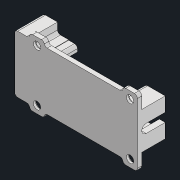
# Autodesk Inventor part: SyringeCasing
Saved by Autodesk Inventor 2022.2 (Build 262287010, 287A)
## iProperties
Created: 2022-06-05
Part Number: SyringeCasing
Material: Generic
Document SubType Name: Modeling
Designer: frede
Density: 1 g/cm^3
Appearance: Default
Author: frede
Autodesk Inventor part; units mm, degrees
ref_plane "YZ Plane" through (0, 0, 0) normal (1, 0, 0) x (0, 1, 0)
ref_plane "XZ Plane" through (0, 0, 0) normal (0, 1, 0) x (-1, 0, 0)
ref_plane "XY Plane" through (0, 0, 0) normal (0, 0, 1) x (1, 0, 0)
sketch "Sketch1" plane through (0, 0, 0) normal (0, 0, 1) x (1, 0, 0)
  line L0 (-75.5, -15.5) -> (-73.5, -15.5) construction
  line L1 (-75.5, 15.5) -> (-73.5, 15.5) construction
  line L2 (-75.5, 15.5) -> (-75.5, 10.4021) construction
  line L3 (-75.5, 10.4021) -> (-75.5, 3.3083) construction
  line L4 (-75.5, 3.3083) -> (-75.5, -3.3083) construction
  line L5 (-75.5, -3.3083) -> (-75.5, -10.4021) construction
  line L6 (-75.5, -10.4021) -> (-75.5, -15.5) construction
  line L7 (-73.5, -15.5) -> (-73.5, -10.4021) construction
  line L8 (-73.5, 10.4021) -> (-73.5, 15.5) construction
  line L9 (-73.5, -8.85) -> (-65.9, -8.85) construction
  line L10 (-73.5, 8.85) -> (-65.9, 8.85) construction
  line L11 (0, 8.575) -> (0, -8.575) construction
  line L12 (0, -8.575) -> (-65.9, -8.575) construction
  line L13 (0, 8.575) -> (-65.9, 8.575) construction
  line L14 (-65.9, 8.575) -> (-65.9, 8.85) construction
  line L15 (-65.9, -8.85) -> (-65.9, -8.575) construction
  line L16 (-73.5, -10.4021) -> (-73.5, -8.85) construction
  line L17 (-73.5, 8.85) -> (-73.5, 10.4021) construction
  line L18 (-65.8, 8.675) -> (0.1, 8.675)
  line L19 (0.1, 8.675) -> (0.1, -8.675)
  line L20 (0.1, -8.675) -> (-65.8, -8.675)
  line L21 (-65.8, -8.675) -> (-65.8, -8.95)
  line L22 (-65.8, -8.95) -> (-73.4, -8.95)
  line L23 (-73.4, -8.95) -> (-73.4, -10.4021)
  line L24 (-73.4, -10.4021) -> (-73.4, -15.6)
  line L25 (-73.4, -15.6) -> (-75.6, -15.6)
  line L26 (-75.6, -15.6) -> (-75.6, -10.4021)
  line L27 (-75.6, -10.4021) -> (-75.6, -3.3083)
  line L28 (-75.6, -3.3083) -> (-75.6, 3.3083)
  line L29 (-75.6, 3.3083) -> (-75.6, 10.4021)
  line L30 (-75.6, 10.4021) -> (-75.6, 15.6)
  line L31 (-75.6, 15.6) -> (-73.4, 15.6)
  line L32 (-73.4, 15.6) -> (-73.4, 10.4021)
  line L33 (-73.4, 10.4021) -> (-73.4, 8.95)
  line L34 (-73.4, 8.95) -> (-65.8, 8.95)
  line L35 (-65.8, 8.95) -> (-65.8, 8.675)
  line L36 (4.1, 12.675) -> (-61.8, 12.675)
  line L37 (-61.8, 12.675) -> (-61.8, 12.95)
  line L38 (-61.8, 12.95) -> (-69.4, 12.95)
  line L39 (-69.4, 12.95) -> (-69.4, 19.6)
  line L40 (-69.4, 19.6) -> (-79.6, 19.6)
  line L41 (-79.6, 19.6) -> (-79.6, 10.4021)
  line L42 (-79.6, 10.4021) -> (-79.6, 3.3083)
  line L43 (-79.6, 3.3083) -> (-79.6, -3.3083)
  line L44 (-79.6, -3.3083) -> (-79.6, -10.4021)
  line L45 (-79.6, -10.4021) -> (-79.6, -19.6)
  line L46 (-79.6, -19.6) -> (-69.4, -19.6)
  line L47 (-69.4, -19.6) -> (-69.4, -12.95)
  line L48 (-69.4, -12.95) -> (-61.8, -12.95)
  line L49 (-61.8, -12.95) -> (-61.8, -12.675)
  line L50 (-61.8, -12.675) -> (4.1, -12.675)
  line L51 (4.1, -12.675) -> (4.1, 12.675)
  dimension "SyringeHolderWallOffset" = 0.1
  dimension "SyringeHolderWallWidth" = 4
  constraints: 88 end point, 6 horizontal, 2 collinear, 2 parallel, 2 vertical, 42 other
  measures "SyringeHolderWallOffset" distance between parallel lines of L13 L18
  measures "SyringeHolderWallWidth" distance between parallel lines of L18 L36
extrude "Extrusion1" add sketch "Sketch1" along normal blind 16
sketch "Sketch2" plane through (0, 0, 16) normal (0, 0, 1) x (1, 0, 0)
  line L0 (-5.9, 19.6) -> (-5.9, 22.675)
  line L1 (-5.9, 22.675) -> (4.1, 22.675)
  line L2 (4.1, 22.675) -> (4.1, 12.675)
  line L3 (-59.4, 19.6) -> (-59.4, 22.675)
  line L4 (-59.4, 22.675) -> (-69.4, 22.675)
  line L5 (-59.4, 19.6) -> (-5.9, 19.6)
  circle A0 centre (-0.9, 17.675) radius 2.5
  circle A1 centre (-64.4, 17.675) radius 2.5
  line L6 (-69.4, 19.6) -> (-79.6, 19.6) projected
  line L7 (-79.6, 19.6) -> (-79.6, -19.6) projected
  line L8 (4.1, -12.675) -> (4.1, 12.675) projected
  line L9 (-69.4, 22.675) -> (-69.4, 19.6)
  line L10 (4.1, 0) -> (-79.6, 0)
  point P0 (-5.9, 21.1375)
  point P1 (4.1, 17.675)
  point P2 (-0.9, 22.675)
  point P3 (-64.4, 22.675)
  dimension "d60" = 10
  dimension "d73" = 5
  constraints: 16 end point, 6 midpoint, 4 horizontal alignment, 4 vertical, 3 horizontal, 2 centre point, 2 equal length, 2 vertical alignment, 1 equal radius
  measures "d60" distance of L0.end L1.end
  measures "d73" diameter of A0
extrude "Extrusion2" add sketch "Sketch2" along normal blind 3
chamfer "Chamfer4" distance 1.5 angle 45 2 edges at (-3.4, 17.675, 16) (-66.9, 17.675, 16)
mirror "Mirror1" about plane through (0, 0, 0) normal (0, 1, 0) of "Extrusion2", "Chamfer4"
sketch "Sketch8" plane through (4.1, -12.675, 0) normal (1, 0, 0) x (0, 0, -1)
  line L0 (0, 0) -> (0, 25.35) construction
  line L1 (0, 15.675) -> (-13, 15.675)
  line L2 (-13, 9.675) -> (0, 9.675)
  line L3 (0, 9.675) -> (0, 15.675)
  arc A0 (-13, 15.675) -> (-13, 9.675) centre (-13, 12.675) ccw
  point P0 (-16, 0)
  point P1 (0, 12.675)
  point P2 (0, 12.675)
  point P3 (-16, 12.675)
  dimension "SyringeHolderTipWidth" = 6
  constraints: 6 end point, 3 point on circle, 2 midpoint, 2 tangent, 1 centre point, 1 horizontal, 1 parallel, 1 point on line, 1 vertical alignment
  measures "SyringeHolderTipWidth" distance of L2.end L1.start
extrude "Extrusion8" cut sketch "Sketch8" against normal up to surface (4 mm away)
sketch "Sketch9" plane through (-79.6, -19.6, 0) normal (-1, 0, 0) x (0, 0, 1)
  line L0 (0, 39.2) -> (0, 0) construction
  line L1 (0, 11.55) -> (8.1, 11.55)
  line L2 (8.1, 27.65) -> (0, 27.65)
  line L3 (0, 27.65) -> (0, 11.55)
  line L4 (8.1, 11.55) -> (16.15, 19.6)
  line L5 (16.15, 19.6) -> (8.1, 27.65)
  point P0 (0, 19.6)
  point P1 (8.1, 11.8)
  point P2 (8.1, 27.4)
  point P3 (15.9, 19.6)
  dimension "d80" = 0.25
  dimension "d81" = 0.25
  dimension "d84" = 0.25
  constraints: 10 end point, 2 vertical alignment, 1 horizontal, 1 parallel, 1 perpendicular, 1 point on line, 3 other
  measures "d80" distance from line of point (8.1, 11.8) L1
  measures "d81" distance from line of point (8.1, 27.4) L2
  measures "d84" distance of point (15.9, 19.6) L4.end
extrude "Extrusion9" cut sketch "Sketch9" against normal up to surface (4 mm away)
sketch "Sketch11" plane through (-69.4, 12.95, 0) normal (0, 1, 0) x (1, 0, 0)
  line L0 (7.6, 0) -> (0, 0) construction
  line L1 (13.6, 0) -> (59.5, 0)
  line L2 (59.5, 0) -> (59.5, -16)
  line L3 (59.5, -16) -> (13.6, -16)
  line L4 (13.6, -16) -> (13.6, 0)
  line L5 (69.5, -13) -> (69.5, 0) construction
  line L6 (3.6, 0) -> (3.6, -16) construction
  point P0 (69.4, 0)
  dimension "d85" = 10
  dimension "d86" = 10
  constraints: 8 end point, 2 parallel, 1 horizontal, 1 perpendicular, 1 point on line
  measures "d85" distance between parallel lines of L5 L2
  measures "d86" distance between parallel lines of L4 L6
extrude "Extrusion10" cut sketch "Sketch11" against normal through all
fillet "Fillet2" radius 2 24 edges at (-69.4, 22.675, 17.5) (-59.4, 22.675, 17.5) (-5.9, 22.675, 17.5) (4.1, 22.675, 17.5) (-5.9, 19.6, 17.5) (-59.4, 19.6, 17.5) (-69.4, 19.6, 17.5) (-79.6, 19.6, 17.5) (-79.6, 19.6, 8) (-79.6, -19.6, 17.5) (-79.6, -19.6, 8) (4.1, -22.675, 17.5) (-5.9, -22.675, 17.5) (-5.9, -19.6, 17.5) (-59.4, -19.6, 17.5) (-59.4, -22.675, 17.5) (-69.4, -19.6, 17.5) (-69.4, -22.675, 17.5) (-9.9, -12.675, 8) (-9.9, 12.675, 8) (-55.8, -12.675, 8) (-55.8, 12.675, 8) (-69.4, -12.95, 8) (-69.4, 12.95, 8)
equation "\"d60\" = ScrewPlateSize"
equation "\"d73\" = ScrewHoleDia"
equation "\"d17\" = ScrewPlateHeight"
equation "\"d74\" = ScrewHoleFillet"
equation "\"d78\" = ScrewPlateHeight"
equation "\"d80\" = d81"
equation "\"d84\" = d81"
equation "\"d82\" = ScrewPlateHeight"
equation "\"d86\" = d85"
equation "\"ScrewPlateSize\" = 10"
equation "\"ScrewHoleDia\" = 5"
equation "\"ScrewPlateHeight\" = 3"
equation "\"ScrewHoleFillet\" = 1.5"
body "Solid1"
